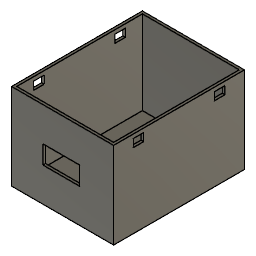
blank-with-usb-slot (Autodesk Fusion 360 design; units mm, degrees)
Autodesk Fusion 360 part; units mm, degrees
sketch "Sketch1" plane through (0, 0, 0) normal (0, 0, 1) x (1, 0, 0)
  line L0 (0, 0) -> (38, 0)
  line L1 (38, 0) -> (38, 50)
  line L2 (38, 50) -> (0, 50)
  line L3 (0, 50) -> (0, 0)
  dimension "d1" = 38
  dimension "d2" = 50
  constraint horizontal L0
  constraint vertical L1
  constraint horizontal L2
  constraint vertical L3
  constraint coincident L0.start L3.end
  measures "d1" distance of L0.start L0.end
  measures "d2" distance of L0.start L2.end
extrude "Extrude1" add sketch "Sketch1" along normal blind 1
extrude "Extrude2" add 1 faces at (12.6667, 33.3333, 1) along direction (0, 0, 1) blind 30 thin wall 1 inside
extrude "Extrude3" add 1 faces at (0.3333, 33, 31) along direction (0, 0, 1) blind 2
sketch "Sketch2" plane through (38, 0, 0) normal (1, 0, 0) x (0, 1, 0)
  line L0 (0, 0) -> (50, 0)
  line L1 (50, 0) -> (50, 33)
  line L2 (50, 33) -> (0, 33)
  line L3 (0, 33) -> (0, 0)
  line L4 (7.5, 32) -> (11.5, 32)
  line L5 (11.5, 32) -> (11.5, 31)
  line L6 (11.5, 31) -> (7.5, 31)
  line L7 (7.5, 31) -> (7.5, 32)
  line L8 (42.5, 32) -> (38.5, 32)
  line L9 (38.5, 32) -> (38.5, 31)
  line L10 (38.5, 31) -> (42.5, 31)
  line L11 (42.5, 31) -> (42.5, 32)
  dimension "d10" = 4
  dimension "d11" = 7.5
  dimension "d12" = 4
  dimension "d13" = 1
  dimension "d14" = 7.5
  constraint horizontal L4
  constraint vertical L5
  constraint horizontal L6
  constraint vertical L7
  constraint horizontal L8
  constraint vertical L9
  constraint horizontal L10
  constraint vertical L11
  measures "d10" distance of L4.start L4.end
  measures "d11" distance of L3 L7
  measures "d12" distance of L8.start L8.end
  measures "d13" distance of L8.start L10.end
  measures "d14" distance of L1 L11
extrude "Extrude4" cut sketch "Sketch2" against normal blind 50 contours L4 L5 L6 L7 | L8 L9 L10 L11
sketch "Sketch3" plane through (0, 0, 0) normal (0, -1, 0) x (1, 0, 0)
  line L0 (0, 0) -> (38, 0)
  line L1 (38, 0) -> (38, 33)
  line L2 (38, 33) -> (0, 33)
  line L3 (0, 33) -> (0, 0)
  line L4 (12, 20) -> (26, 20)
  line L5 (26, 20) -> (26, 13)
  line L6 (26, 13) -> (12, 13)
  line L7 (12, 13) -> (12, 20)
  dimension "d17" = 14
  dimension "d18" = 7
  dimension "d19" = 12
  dimension "d20" = 13
  constraint horizontal L4
  constraint vertical L5
  constraint horizontal L6
  constraint vertical L7
  measures "d17" distance of L4.start L4.end
  measures "d18" distance of L4.start L6.end
  measures "d19" distance of L3 L7
  measures "d20" distance of L2 L4
extrude "Extrude5" cut sketch "Sketch3" against normal blind 2 contours L4 L5 L6 L7
move_face "OffsetFaces1" offset -2.5 4 faces at (0.6667, 10.1667, 31) (0.6667, 39.8333, 31) (37.6667, 39.8333, 31) (37.6667, 10.1667, 31)
move_face "OffsetFaces2" offset 0.5 4 faces at (37.6667, 41.1667, 32) (37.6667, 8.8333, 32) (0.6667, 8.8333, 32) (0.6667, 41.1667, 32)
extrude "Extrude6" add 1 faces at (38, 20.5, 9.5) along direction (1, 0, 0) blind 1
extrude "Extrude7" cut 1 faces at (37, 20.5, 10.1667) along direction (1, 0, 0) blind 1
